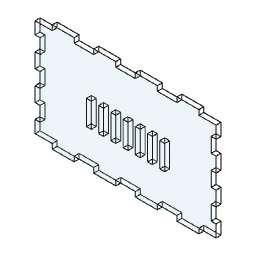
case_6_2mm (Autodesk Fusion 360 design; units mm, degrees)
Autodesk Fusion 360 part; units mm, degrees
sketch "スケッチ1" plane through (0, 0, 0) normal (0, 1, 0) x (1, 0, 0)
  line L0 (0, 0) -> (74, 0)
  line L1 (74, 0) -> (74, -44)
  line L2 (74, -44) -> (0, -44)
  line L3 (0, -44) -> (0, 0)
  dimension "d1" = 74
  dimension "d2" = 44
  constraint horizontal L0
  constraint vertical L1
  constraint horizontal L2
  constraint vertical L3
  constraint coincident L0.start L3.end
  measures "d1" distance of L0.start L0.end
  measures "d2" distance of L0.start L2.end
extrude "押し出し1" add sketch "スケッチ1" along normal blind 2
sketch "スケッチ2" plane through (0, 0, 0) normal (0, -1, 0) x (1, 0, 0)
  line L0 (74, 44) -> (0, 44)
  line L1 (0, 44) -> (0, 0)
  line L2 (0, 0) -> (74, 0)
  line L3 (74, 0) -> (74, 44)
  line L4 (0, 44) -> (7, 44)
  line L5 (7, 44) -> (7, 42)
  line L6 (7, 42) -> (0, 42)
  line L7 (0, 42) -> (0, 44)
  line L8 (16, 42) -> (24, 42)
  line L9 (24, 42) -> (24, 44)
  line L10 (24, 44) -> (16, 44)
  line L11 (16, 44) -> (16, 42)
  line L12 (41, 44) -> (33, 44)
  line L13 (33, 42) -> (41, 42)
  line L14 (41, 42) -> (41, 44)
  line L15 (33, 44) -> (33, 42)
  line L16 (58, 44) -> (50, 44)
  line L17 (50, 42) -> (58, 42)
  line L18 (58, 42) -> (58, 44)
  line L19 (50, 44) -> (50, 42)
  line L20 (67, 42) -> (74, 42)
  line L21 (74, 42) -> (74, 44)
  line L22 (74, 44) -> (67, 44)
  line L23 (67, 44) -> (67, 42)
  line L24 (50, 2) -> (50, 0)
  line L25 (67, 2) -> (67, 0)
  line L26 (16, 0) -> (24, 0)
  line L27 (50, 0) -> (58, 0)
  line L28 (0, 2) -> (7, 2)
  line L29 (67, 0) -> (74, 0)
  line L30 (58, 0) -> (58, 2)
  line L31 (24, 2) -> (16, 2)
  line L32 (33, 2) -> (33, 0)
  line L33 (58, 2) -> (50, 2)
  line L34 (33, 0) -> (41, 0)
  line L35 (0, 0) -> (0, 2)
  line L36 (24, 0) -> (24, 2)
  line L37 (74, 2) -> (67, 2)
  line L38 (7, 2) -> (7, 0)
  line L39 (41, 0) -> (41, 2)
  line L40 (16, 2) -> (16, 0)
  line L41 (74, 0) -> (74, 2)
  line L42 (7, 0) -> (0, 0)
  line L43 (41, 2) -> (33, 2)
  dimension "d5" = 7
  dimension "d6" = 2
  dimension "d7" = 2
  dimension "d8" = 8
  dimension "d9" = 9
  dimension "d12" = 17
  dimension "d13" = 0
  dimension "d14" = 7
  dimension "d15" = 2
  dimension "d16" = 9
  constraint horizontal L4
  constraint vertical L5
  constraint horizontal L6
  constraint vertical L7
  constraint coincident L0.end L1.start
  constraint horizontal L8
  constraint vertical L9
  constraint horizontal L10
  constraint vertical L11
  constraint coincident L0 L9.end
  constraint horizontal L20
  constraint vertical L21
  constraint horizontal L22
  constraint vertical L23
  constraint coincident L0.start L3.end
  measures "d5" distance of L5.end L6.end
  measures "d6" distance of L0.end L6.end
  measures "d7" distance of L8.start L10.end
  measures "d8" distance of L8.start L8.end
  measures "d9" distance of L5 L11
  measures "d14" distance of L0.start L22.end
  measures "d15" distance of L20.end L0.start
  measures "d16" distance of L18 L23
extrude "押し出し2" cut sketch "スケッチ2" against normal blind 2 contours L0 L3 L20 L21 L22 L23 | L0 L16 L17 L18 L19 | L2 L3 L25 L29 L37 L41 | L0 L12 L13 L14 L15 | L2 L24 L27 L30 L33 | L0 L8 L9 L10 L11 | L2 L32 L34 L39 L43 | L0 L1 L4 L5 L6 L7 | L2 L26 L31 L36 L40 | L1 L2 L28 L35 L38 L42
sketch "スケッチ3" plane through (0, 0, 0) normal (0, -1, 0) x (1, 0, 0)
  line L0 (33, 42) -> (33, 44)
  line L1 (33, 44) -> (24, 44)
  line L2 (24, 44) -> (24, 42)
  line L3 (24, 42) -> (16, 42)
  line L4 (16, 42) -> (16, 44)
  line L5 (16, 44) -> (7, 44)
  line L6 (7, 44) -> (7, 42)
  line L7 (7, 42) -> (0, 42)
  line L8 (0, 42) -> (0, 2)
  line L9 (0, 2) -> (7, 2)
  line L10 (7, 2) -> (7, 0)
  line L11 (7, 0) -> (16, 0)
  line L12 (16, 0) -> (16, 2)
  line L13 (16, 2) -> (24, 2)
  line L14 (24, 2) -> (24, 0)
  line L15 (24, 0) -> (33, 0)
  line L16 (33, 0) -> (33, 2)
  line L17 (33, 2) -> (41, 2)
  line L18 (41, 2) -> (41, 0)
  line L19 (41, 0) -> (50, 0)
  line L20 (50, 0) -> (50, 2)
  line L21 (50, 2) -> (58, 2)
  line L22 (58, 2) -> (58, 0)
  line L23 (58, 0) -> (67, 0)
  line L24 (67, 0) -> (67, 2)
  line L25 (67, 2) -> (74, 2)
  line L26 (74, 2) -> (74, 42)
  line L27 (74, 42) -> (67, 42)
  line L28 (67, 42) -> (67, 44)
  line L29 (67, 44) -> (58, 44)
  line L30 (58, 44) -> (58, 42)
  line L31 (58, 42) -> (50, 42)
  line L32 (50, 42) -> (50, 44)
  line L33 (50, 44) -> (41, 44)
  line L34 (41, 44) -> (41, 42)
  line L35 (41, 42) -> (33, 42)
  line L36 (2, 37) -> (0, 37)
  line L37 (0, 37) -> (0, 31)
  line L38 (0, 31) -> (2, 31)
  line L39 (2, 31) -> (2, 37)
  line L40 (0, 19) -> (2, 19)
  line L41 (0, 25) -> (0, 19)
  line L42 (2, 25) -> (0, 25)
  line L43 (2, 19) -> (2, 25)
  line L44 (0, 7) -> (2, 7)
  line L45 (0, 13) -> (0, 7)
  line L46 (2, 13) -> (0, 13)
  line L47 (2, 7) -> (2, 13)
  line L48 (72, 31) -> (74, 31)
  line L49 (74, 37) -> (72, 37)
  line L50 (74, 25) -> (72, 25)
  line L51 (72, 37) -> (72, 31)
  line L52 (72, 19) -> (74, 19)
  line L53 (72, 7) -> (74, 7)
  line L54 (74, 19) -> (74, 25)
  line L55 (72, 25) -> (72, 19)
  line L56 (74, 7) -> (74, 13)
  line L57 (74, 31) -> (74, 37)
  line L58 (72, 13) -> (72, 7)
  line L59 (74, 13) -> (72, 13)
  dimension "d23" = 7
  dimension "d24" = 6
  dimension "d25" = 2
  dimension "d28" = 0
  dimension "d29" = -12
  dimension "d30" = 7
  dimension "d33" = 72
  dimension "d34" = 0
  constraint horizontal L36
  constraint vertical L37
  constraint horizontal L38
  constraint vertical L39
  constraint coincident L8 L37.end
  measures "d23" distance of L5 L36
  measures "d24" distance of L36.start L38.end
  measures "d25" distance of L36.start L36.end
  measures "d30" distance of L11 L44
extrude "押し出し3" cut sketch "スケッチ3" against normal blind 2 contours L8 L36 L37 L38 L39 | L26 L48 L49 L51 L57 | L8 L40 L41 L42 L43 | L26 L50 L52 L54 L55 | L8 L44 L45 L46 L47 | L26 L53 L56 L58 L59
sketch "スケッチ4" plane through (0, 0, 0) normal (0, -1, 0) x (1, 0, 0)
  line L0 (2, 31) -> (0, 31)
  line L1 (0, 31) -> (0, 25)
  line L2 (0, 25) -> (2, 25)
  line L3 (2, 25) -> (2, 19)
  line L4 (2, 19) -> (0, 19)
  line L5 (0, 19) -> (0, 13)
  line L6 (0, 13) -> (2, 13)
  line L7 (2, 13) -> (2, 7)
  line L8 (2, 7) -> (0, 7)
  line L9 (0, 7) -> (0, 2)
  line L10 (0, 2) -> (7, 2)
  line L11 (7, 2) -> (7, 0)
  line L12 (7, 0) -> (16, 0)
  line L13 (16, 0) -> (16, 2)
  line L14 (16, 2) -> (24, 2)
  line L15 (24, 2) -> (24, 0)
  line L16 (24, 0) -> (33, 0)
  line L17 (33, 0) -> (33, 2)
  line L18 (33, 2) -> (41, 2)
  line L19 (41, 2) -> (41, 0)
  line L20 (41, 0) -> (50, 0)
  line L21 (50, 0) -> (50, 2)
  line L22 (50, 2) -> (58, 2)
  line L23 (58, 2) -> (58, 0)
  line L24 (58, 0) -> (67, 0)
  line L25 (67, 0) -> (67, 2)
  line L26 (67, 2) -> (74, 2)
  line L27 (74, 2) -> (74, 7)
  line L28 (74, 7) -> (72, 7)
  line L29 (72, 7) -> (72, 13)
  line L30 (72, 13) -> (74, 13)
  line L31 (74, 13) -> (74, 19)
  line L32 (74, 19) -> (72, 19)
  line L33 (72, 19) -> (72, 25)
  line L34 (72, 25) -> (74, 25)
  line L35 (74, 25) -> (74, 31)
  line L36 (74, 31) -> (72, 31)
  line L37 (72, 31) -> (72, 37)
  line L38 (72, 37) -> (74, 37)
  line L39 (74, 37) -> (74, 42)
  line L40 (74, 42) -> (67, 42)
  line L41 (67, 42) -> (67, 44)
  line L42 (67, 44) -> (58, 44)
  line L43 (58, 44) -> (58, 42)
  line L44 (58, 42) -> (50, 42)
  line L45 (50, 42) -> (50, 44)
  line L46 (50, 44) -> (41, 44)
  line L47 (41, 44) -> (41, 42)
  line L48 (41, 42) -> (33, 42)
  line L49 (33, 42) -> (33, 44)
  line L50 (33, 44) -> (24, 44)
  line L51 (24, 44) -> (24, 42)
  line L52 (24, 42) -> (16, 42)
  line L53 (16, 42) -> (16, 44)
  line L54 (16, 44) -> (7, 44)
  line L55 (7, 44) -> (7, 42)
  line L56 (7, 42) -> (0, 42)
  line L57 (0, 42) -> (0, 37)
  line L58 (0, 37) -> (2, 37)
  line L59 (2, 37) -> (2, 31)
  line L60 (36, 15) -> (38, 15)
  line L61 (38, 15) -> (38, 25)
  line L62 (38, 25) -> (36, 25)
  line L63 (36, 25) -> (36, 15)
  line L64 (33, 15) -> (31, 15)
  line L65 (31, 15) -> (31, 25)
  line L66 (31, 25) -> (33, 25)
  line L67 (33, 25) -> (33, 15)
  line L68 (28, 15) -> (26, 15)
  line L69 (26, 15) -> (26, 25)
  line L70 (26, 25) -> (28, 25)
  line L71 (28, 25) -> (28, 15)
  line L72 (41, 15) -> (43, 15)
  line L73 (43, 15) -> (43, 25)
  line L74 (43, 25) -> (41, 25)
  line L75 (41, 25) -> (41, 15)
  line L76 (46, 15) -> (48, 15)
  line L77 (48, 15) -> (48, 25)
  line L78 (48, 25) -> (46, 25)
  line L79 (46, 25) -> (46, 15)
  line L80 (23, 15) -> (21, 15)
  line L81 (21, 15) -> (21, 25)
  line L82 (21, 25) -> (23, 25)
  line L83 (23, 25) -> (23, 15)
  line L84 (51, 15) -> (53, 15)
  line L85 (53, 15) -> (53, 25)
  line L86 (53, 25) -> (51, 25)
  line L87 (51, 25) -> (51, 15)
  constraint horizontal L60
  constraint vertical L61
  constraint horizontal L62
  constraint vertical L63
  constraint horizontal L64
  constraint vertical L65
  constraint horizontal L66
  constraint vertical L67
  constraint horizontal L68
  constraint vertical L69
  constraint horizontal L70
  constraint vertical L71
  constraint horizontal L72
  constraint vertical L73
  constraint horizontal L74
  constraint vertical L75
  constraint horizontal L76
  constraint vertical L77
  constraint horizontal L78
  constraint vertical L79
  constraint horizontal L80
  constraint vertical L81
  constraint horizontal L82
  constraint vertical L83
  constraint horizontal L84
  constraint vertical L85
  constraint horizontal L86
  constraint vertical L87
extrude "押し出し4" cut sketch "スケッチ4" against normal blind 2 contours L60 L61 L62 L63 | L64 L65 L66 L67 | L68 L69 L70 L71 | L72 L73 L74 L75 | L76 L77 L78 L79 | L80 L81 L82 L83 | L84 L85 L86 L87
sketch "スケッチ5" plane through (0, 0, 0) normal (0, -1, 0) x (1, 0, 0)
  line L0 (31, 15) -> (31, 25)
  line L1 (31, 25) -> (33, 25)
  line L2 (33, 25) -> (33, 15)
  line L3 (33, 15) -> (31, 15)
  line L4 (38, 15) -> (36, 15)
  line L5 (36, 15) -> (36, 25)
  line L6 (36, 25) -> (38, 25)
  line L7 (38, 25) -> (38, 15)
  line L8 (26, 15) -> (26, 25)
  line L9 (26, 25) -> (28, 25)
  line L10 (28, 25) -> (28, 15)
  line L11 (28, 15) -> (26, 15)
  line L12 (21, 15) -> (21, 25)
  line L13 (21, 25) -> (23, 25)
  line L14 (23, 25) -> (23, 15)
  line L15 (23, 15) -> (21, 15)
  line L16 (48, 15) -> (46, 15)
  line L17 (46, 15) -> (46, 25)
  line L18 (46, 25) -> (48, 25)
  line L19 (48, 25) -> (48, 15)
  line L20 (43, 15) -> (41, 15)
  line L21 (41, 15) -> (41, 25)
  line L22 (41, 25) -> (43, 25)
  line L23 (43, 25) -> (43, 15)
  line L24 (53, 15) -> (51, 15)
  line L25 (51, 15) -> (51, 25)
  line L26 (51, 25) -> (53, 25)
  line L27 (53, 25) -> (53, 15)
  line L28 (2, 31) -> (0, 31)
  line L29 (0, 31) -> (0, 25)
  line L30 (0, 25) -> (2, 25)
  line L31 (2, 25) -> (2, 19)
  line L32 (2, 19) -> (0, 19)
  line L33 (0, 19) -> (0, 13)
  line L34 (0, 13) -> (2, 13)
  line L35 (2, 13) -> (2, 7)
  line L36 (2, 7) -> (0, 7)
  line L37 (0, 7) -> (0, 2)
  line L38 (0, 2) -> (7, 2)
  line L39 (7, 2) -> (7, 0)
  line L40 (7, 0) -> (16, 0)
  line L41 (16, 0) -> (16, 2)
  line L42 (16, 2) -> (24, 2)
  line L43 (24, 2) -> (24, 0)
  line L44 (24, 0) -> (33, 0)
  line L45 (33, 0) -> (33, 2)
  line L46 (33, 2) -> (41, 2)
  line L47 (41, 2) -> (41, 0)
  line L48 (41, 0) -> (50, 0)
  line L49 (50, 0) -> (50, 2)
  line L50 (50, 2) -> (58, 2)
  line L51 (58, 2) -> (58, 0)
  line L52 (58, 0) -> (67, 0)
  line L53 (67, 0) -> (67, 2)
  line L54 (67, 2) -> (74, 2)
  line L55 (74, 2) -> (74, 7)
  line L56 (74, 7) -> (72, 7)
  line L57 (72, 7) -> (72, 13)
  line L58 (72, 13) -> (74, 13)
  line L59 (74, 13) -> (74, 19)
  line L60 (74, 19) -> (72, 19)
  line L61 (72, 19) -> (72, 25)
  line L62 (72, 25) -> (74, 25)
  line L63 (74, 25) -> (74, 31)
  line L64 (74, 31) -> (72, 31)
  line L65 (72, 31) -> (72, 37)
  line L66 (72, 37) -> (74, 37)
  line L67 (74, 37) -> (74, 42)
  line L68 (74, 42) -> (67, 42)
  line L69 (67, 42) -> (67, 44)
  line L70 (67, 44) -> (58, 44)
  line L71 (58, 44) -> (58, 42)
  line L72 (58, 42) -> (50, 42)
  line L73 (50, 42) -> (50, 44)
  line L74 (50, 44) -> (41, 44)
  line L75 (41, 44) -> (41, 42)
  line L76 (41, 42) -> (33, 42)
  line L77 (33, 42) -> (33, 44)
  line L78 (33, 44) -> (24, 44)
  line L79 (24, 44) -> (24, 42)
  line L80 (24, 42) -> (16, 42)
  line L81 (16, 42) -> (16, 44)
  line L82 (16, 44) -> (7, 44)
  line L83 (7, 44) -> (7, 42)
  line L84 (7, 42) -> (0, 42)
  line L85 (0, 42) -> (0, 37)
  line L86 (0, 37) -> (2, 37)
  line L87 (2, 37) -> (2, 31)
